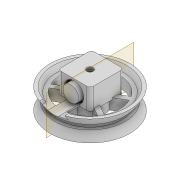
# Autodesk Inventor part: Primary_hinge
Saved by Autodesk Inventor 2022 (Build 260153000, 153)
## iProperties
Created: 2022-07-14
Part Number: Primary_hinge
Material: Generic
Document SubType Name: Modeling
Designer: dell
Density: 1 g/cm^3
Appearance: Default
Mass: 11.9893 g
Surface Area: 101.14 cm^2
Volume: 11.9893 cm^3
Author: dell
Autodesk Inventor part; units mm, degrees
ref_plane "XZ Plane" through (0, 0, 0) normal (0, 1, 0) x (-1, 0, 0)
ref_plane "XY Plane" through (0, 0, 0) normal (0, 0, 1) x (1, 0, 0)
sketch "Sketch1" plane through (0, 0, 0) normal (0, 0, 1) x (1, 0, 0)
  circle A0 centre (0, 0) radius 4.9
  circle A1 centre (0, 0) radius 6.1
  line L0 (-10.1, -7.1) -> (10.1, -7.1)
  line L1 (10.1, -7.1) -> (10.1, 7.1)
  line L2 (10.1, 7.1) -> (-10.1, 7.1)
  line L3 (-10.1, 7.1) -> (-10.1, -7.1)
  line L4 (-10.1, -7.1) -> (10.1, 7.1) construction
  line L5 (10.1, -7.1) -> (-10.1, 7.1) construction
  dimension "d0" = 9.8
  dimension "d1" = 12.2
  dimension "d3" = 4
  dimension "d4" = 1
  constraints: 12 end point, 2 centre point, 2 coincident, 2 midpoint, 2 parallel, 1 horizontal, 1 perpendicular
  measures "d0" diameter of A0
  measures "d1" diameter of A1
  measures "d3" distance edge to line of A1 L1
  measures "d4" distance edge to line of A1 L2
extrude "Extrusion1" add sketch "Sketch1" along normal blind 18
sketch "Sketch2" plane through (0, 0, 18) normal (0, 0, 1) x (1, 0, 0)
  circle A0 centre (0, 0) radius 4.9 projected
extrude "Extrusion2" add sketch "Sketch2" along normal blind 2
sketch "Sketch3" plane through (0, 0, 0) normal (0, 0, -1) x (-1, 0, 0)
  line L0 (-10.1, -7.1) -> (-10.1, 7.1) projected
  line L1 (10.1, -7.1) -> (-10.1, -7.1) projected
  line L2 (10.1, 7.1) -> (10.1, -7.1) projected
  line L3 (-10.1, 7.1) -> (10.1, 7.1) projected
  circle A0 centre (0, 0) radius 6.1 projected
extrude "Extrusion3" add sketch "Sketch3" along normal blind 3 contours L0 L3 L2 L1 | A0
ref_plane "Work Plane1" through (0, -7.1, 18) normal (-1, 0, 0) x (0, 0, 1)
sketch "Sketch6" plane through (-10.1, 7.1, 18) normal (0, 1, 0) x (1, 0, 0)
  line L0 (5.2, 18) -> (15, 18) projected
  line L1 (16.2, 18) -> (4, 18) projected
  line L2 (20.2, 0) -> (0, 0) projected
  line L3 (0, 21) -> (20.2, 21) projected
  line L4 (16.2, 0) -> (16.2, 18) projected
  line L5 (4, 0) -> (4, 18) projected
  circle A0 centre (10.1, 10) radius 2.05
  line L6 (0, 21) -> (0, 0) projected
  line L7 (20.2, 21) -> (20.2, 0) projected
  point P0 (10.1, 18)
  point P1 (10.1, 18)
  dimension "d49" = 4.1
  dimension "d50" = 10
  constraints: 1 centre point, 1 coincident, 1 midpoint, 1 vertical alignment
  measures "d49" diameter of A0
  measures "d50" distance from line of L2 A0.centre
extrude "Extrusion12" cut sketch "Sketch6" against normal blind 100 contours A0
fillet "Fillet5" radius 2 4 edges at (10.1, 0, 18) (-10.1, 0, 18) (10.1, 0, -3) (-10.1, 0, -3)
sketch "Sketch14" plane through (-8.1, -7.1, -3) normal (0, -1, 0) x (1, 0, 0)
  circle A0 centre (8.1, 11) radius 2.05 projected
  line L0 (8.1, 15.0415) -> (11.6, 13.0207)
  line L1 (11.6, 13.0207) -> (11.6, 8.9793)
  line L2 (11.6, 8.9793) -> (8.1, 6.9585)
  line L3 (8.1, 6.9585) -> (4.6, 8.9793)
  line L4 (4.6, 8.9793) -> (4.6, 13.0207)
  line L5 (4.6, 13.0207) -> (8.1, 15.0415)
  circle A1 centre (8.1, 11) radius 8
  point P0 (8.1, 3)
  dimension "d69" = 7
  dimension "d73" = 16
  constraints: 12 end point, 2 coincident, 1 centre point, 13 other
  measures "d69" distance between parallel lines of L1 L4
  measures "d73" diameter of A1
extrude "Extrusion14" add sketch "Sketch14" along normal blind 5 contours A1
sketch "Sketch15" plane through (0, -12.1, 8) normal (0, -1, 0) x (1, 0, 0)
  line L0 (3.4, -1) -> (4.8, -1)
  line L1 (4.8, -1) -> (4.8, -7.2415)
  line L2 (4.8, -7.2415) -> (3.4, -7.2415)
  line L3 (3.4, -7.2415) -> (3.4, -1)
  line L4 (3.4, -1) -> (4.8, -7.2415) construction
  line L5 (4.8, -1) -> (3.4, -7.2415) construction
  line L6 (0, 16.6) -> (0, -15.6) projected
  circle A0 centre (0, 0) radius 2.05 projected
  circle A1 centre (0, 0) radius 4.5
  circle A2 centre (0, 0) radius 8 projected
  line L7 (0, 4.0415) -> (3.5, 2.0207) projected
  line L8 (3.5, 2.0207) -> (3.5, -2.0207) projected
  line L9 (3.5, -2.0207) -> (0, -4.0415) projected
  line L10 (0, -4.0415) -> (-3.5, -2.0207) projected
  line L11 (-3.5, -2.0207) -> (-3.5, 2.0207) projected
  line L12 (-3.5, 2.0207) -> (0, 4.0415) projected
  circle A3 centre (0, 0) radius 8 projected
  line L13 (1.4, -7.8765) -> (3.4, -7.8765)
  line L14 (3.4, -7.8765) -> (3.4, -4.8765)
  line L15 (3.4, -4.8765) -> (1.4, -4.8765)
  line L16 (1.4, -4.8765) -> (1.4, -7.8765)
  line L17 (4.8, -6.4) -> (6.8, -6.4)
  line L18 (6.8, -6.4) -> (6.8, -2.4)
  line L19 (6.8, -2.4) -> (4.8, -2.4)
  line L20 (4.8, -2.4) -> (4.8, -6.4)
  line L21 (4.8, 1) -> (3.4, 1)
  line L22 (3.4, 1) -> (3.4, 7.2415)
  line L23 (3.4, 7.2415) -> (4.8, 7.2415)
  line L24 (4.8, 7.2415) -> (4.8, 1)
  line L25 (4.8, 1) -> (3.4, 7.2415) construction
  line L26 (3.4, 1) -> (4.8, 7.2415) construction
  line L27 (4.8, 6.4) -> (6.8, 6.4)
  line L28 (6.8, 6.4) -> (6.8, 3.4)
  line L29 (6.8, 3.4) -> (4.8, 3.4)
  line L30 (4.8, 3.4) -> (4.8, 6.4)
  line L31 (1.4, 8.7415) -> (3.4, 8.7415)
  line L32 (3.4, 8.7415) -> (3.4, 5.7415)
  line L33 (3.4, 5.7415) -> (1.4, 5.7415)
  line L34 (1.4, 5.7415) -> (1.4, 8.7415)
  point P0 (0, -8)
  point P1 (4.1, -4.1208)
  point P2 (4.8, -6.4)
  point P3 (6.8, -4.2143)
  point P4 (4.1, 4.1208)
  point P5 (4.8, 3.4)
  point P6 (6.8, 4.2143)
  point P7 (4.8, 6.4)
  point P8 (1.4, 7.8765)
  point P9 (4.8, 6.4)
  dimension "d74" = 4.1
  dimension "d75" = 1.4
  dimension "d76" = 9
  dimension "d77" = 1
  dimension "d78" = 2
  dimension "d79" = 3
  dimension "d80" = 2
  dimension "d81" = 4
  dimension "d84" = 1.4
  dimension "d85" = 1
  dimension "d86" = 4.1
  dimension "d87" = 2
  dimension "d88" = 3
  dimension "d89" = 2
  dimension "d90" = 3
  dimension "d97" = 1.5
  constraints: 56 end point, 12 parallel, 6 horizontal, 6 perpendicular, 4 midpoint, 4 point on circle, 4 point on line, 1 centre point, 1 coincident, 3 other
  measures "d74" distance from line of L6 point (4.1, -4.121)
  measures "d75" distance between parallel lines of L1 L3
  measures "d76" diameter of A1
  measures "d77" distance from line of A0.centre L0
  measures "d78" distance between parallel lines of L14 L16
  measures "d79" distance between parallel lines of L13 L15
  measures "d80" distance between parallel lines of L1 L18
  measures "d81" distance between parallel lines of L17 L19
  measures "d84" distance between parallel lines of L22 L24
  measures "d85" distance from line of A0.centre L21
  measures "d86" horizontal distance of A0.centre point (4.1, 4.121)
  measures "d87" distance of L28.end L29.end
  measures "d88" distance of L27.end L28.end
  measures "d89" distance of L31.start L31.end
  measures "d90" distance of L33.end L31.start
  measures "d97" distance between parallel lines of L23 L31
extrude "Extrusion15" add sketch "Sketch15" along normal blind 3 contours L33 L34 A2 L22 | L24 A2 L28 L29 | A2 L34 L31 L32 | L27 L28 A2
sketch "Sketch16" plane through (-3.5, -7.1, 5.9793) normal (0, -1, 0) x (1, 0, 0)
  line L0 (3.5, 6.0622) -> (0, 4.0415) projected
  line L1 (0, 4.0415) -> (0, 0) projected
  line L2 (0, 0) -> (3.5, -2.0207) projected
  line L3 (3.5, -2.0207) -> (7, 0) projected
  line L4 (7, 0) -> (7, 4.0415) projected
  line L5 (7, 4.0415) -> (3.5, 6.0622) projected
  circle A0 centre (3.5, 2.0207) radius 2.05 projected
  point P0 (3.5, -5.9793)
extrude "Extrusion16" add sketch "Sketch16" along normal blind 2.4
sketch "Sketch17" plane through (-8.1, -12.1, -3) normal (0, -1, 0) x (1, 0, 0)
  arc A0 (12.9, 17.4) -> (11.5, 18.2415) centre (8.1, 11) ccw projected
  circle A1 centre (8.1, 11) radius 25
  circle A2 centre (8.1, 11) radius 8
  point P0 (8.1, 3)
  point P1 (9.5, 18.8765)
  point P2 (9.5, 18.8765)
  point P3 (14.9, 15.2143)
  dimension "d94" = 17
  constraints: 2 centre point, 2 coincident, 1 concentric
  measures "d94" radial gap between concentric circles of A0 A1
extrude "Extrusion17" add sketch "Sketch17" against normal blind 2
sketch "Sketch19" plane through (0, 0, 18) normal (0, 0, 1) x (1, 0, 0)
  circle A0 centre (0, 0) radius 4.9 projected
  circle A1 centre (0, 0) radius 6.1 projected
  circle A2 centre (0, 0) radius 4.9 projected
sketch "Sketch18" plane through (-8.1, -7.1, -3) normal (0, -1, 0) x (1, 0, 0)
  circle A0 centre (8.1, 11) radius 25 projected
  arc A1 (-2, 2) -> (0, 0) centre (0, 2) ccw projected
  line L0 (16.2, 0) -> (0, 0) projected
  arc A2 (16.2, 0) -> (18.2, 2) centre (16.2, 2) ccw projected
  line L1 (18.2, 19) -> (18.2, 2) projected
  arc A3 (18.2, 19) -> (16.2, 21) centre (16.2, 19) ccw projected
  line L2 (0, 21) -> (16.2, 21) projected
  arc A4 (0, 21) -> (-2, 19) centre (0, 19) ccw projected
  line L3 (-2, 2) -> (-2, 19) projected
  circle A5 centre (8.1, 11) radius 8 projected
  point P0 (8.1, 3)
extrude "Extrusion18" add sketch "Sketch18" against normal blind 2 contours A0
extrude "Extrusion19" cut sketch "Sketch19" along normal blind 100
thicken "Thicken1" operation add thickness 12 both sides no extend neighbours yes toward (0.9967573, 0, -0.0804666) faces at (7.9741, -8.1, 7.3563)
sketch "Sketch20" plane through (0, -12.1, 8) normal (0, -1, 0) x (1, 0, 0)
  circle A0 centre (0, 0) radius 25 projected
  circle A1 centre (0, 0) radius 21
  point P0 (0, -8)
  dimension "d104" = 4
  constraints: 1 centre point
  measures "d104" radial gap between concentric circles of A0 A1
extrude "Extrusion20" add sketch "Sketch20" along normal blind 3
sketch "Sketch21" plane through (-8.1, -5.1, -3) normal (0, 1, 0) x (1, 0, 0)
  arc A0 (11.4466, -35.775) -> (4.7534, -35.775) centre (8.1, -11) ccw projected
  arc A1 (11.1556, -31.7765) -> (5.0444, -31.7765) centre (8.1, -11) ccw
  circle A2 centre (8.1, -11) radius 2.05 projected
  circle A3 centre (8.1, -11) radius 21
  circle A4 centre (8.1, -11) radius 21 projected
  line L0 (0.1, -30.4165) -> (0.1, -34.6854)
  line L1 (16.1, -30.4165) -> (16.1, -34.6854)
  point P0 (8.1, -3)
  point P1 (11.4466, -33.7552)
  point P2 (4.7534, -33.7552)
  point P3 (16.1, -30.4165)
  point P4 (18.1, -31.7123)
  point P5 (-1.9, -31.7123)
  point P6 (0.1, -30.4165)
  dimension "d107" = 4
  dimension "d108" = 8
  dimension "d109" = 8
  constraints: 6 point on circle, 4 end point, 2 centre point, 1 coincident, 1 concentric, 1 parallel, 1 vertical
  measures "d107" radial gap between concentric circles of A0 A1
  measures "d108" distance from line of A0.centre L1
  measures "d109" distance from line of A0.centre L0
extrude "Extrusion21" add sketch "Sketch21" along normal blind 3 contours L1 A1 L0 A0
chamfer "Chamfer1" distance 3 distance2 5 1 edges at (-25, -7.1, 8) measured on face at (-24.5, -7.1, 8)
chamfer "Chamfer2" distance 3 distance2 5 1 edges at (-25, -10.1, 8) measured on face at (-24.5, -10.1, 8)
chamfer "Chamfer3" distance 2 distance2 3 1 edges at (0, -2.1, -13) measured on face at (0, -2.1, -13.5)
chamfer "Chamfer4" distance 2 distance2 3 1 edges at (-21, -15.1, 8) measured on face at (-21.5, -15.1, 8)
sketch "Sketch22" plane through (0, -12.1, 8) normal (0, -1, 0) x (1, 0, 0)
  circle A0 centre (0.0592, 0.0061) radius 18.5
  circle A1 centre (0.0592, 0.0061) radius 9.5
  line L0 (-1.5, 18.4403) -> (-1.5, -18.4281)
  line L1 (1.5, -18.4377) -> (1.5, 18.4499)
  line L2 (0, 35) -> (0, -35) projected
  line L3 (-15.1257, -10.5613) -> (16.8033, 7.8729)
  line L4 (15.3116, 10.4758) -> (-16.634, -7.9681)
  line L5 (16.8033, -7.8607) -> (-15.1257, 10.5735)
  line L6 (-16.634, 7.9802) -> (15.3116, -10.4636)
  arc A2 (8, 21.7771) -> (3.3466, 22.9574) centre (0, 0) ccw projected
  line L7 (8, 21.7771) -> (8, 19.4165) projected
  arc A3 (-8, 19.4165) -> (8, 19.4165) centre (0, 0) ccw projected
  line L8 (-8, 19.4165) -> (-8, 21.7771) projected
  arc A4 (-3.3466, 22.9574) -> (-8, 21.7771) centre (0, 0) ccw projected
  line L9 (-3.3466, 22.9574) -> (-3.3466, 10) projected
  line L10 (-8.1, 10) -> (-3.3466, 10) projected
  arc A5 (-8.1, 10) -> (-10.1, 8) centre (-8.1, 8) ccw projected
  line L11 (-10.1, -9) -> (-10.1, 8) projected
  arc A6 (-10.1, -9) -> (-8.1, -11) centre (-8.1, -9) ccw projected
  line L12 (8.1, -11) -> (-8.1, -11) projected
  arc A7 (8.1, -11) -> (10.1, -9) centre (8.1, -9) ccw projected
  line L13 (10.1, 8) -> (10.1, -9) projected
  arc A8 (10.1, 8) -> (8.1, 10) centre (8.1, 8) ccw projected
  line L14 (3.3466, 10) -> (8.1, 10) projected
  line L15 (3.3466, 10) -> (3.3466, 22.9574) projected
  point P0 (0, -8)
  point P1 (16.8033, -7.8607)
  point P2 (-1.5, -9.3651)
  point P3 (8.9545, -3.3292)
  point P4 (15.3116, -10.4636)
  point P5 (7.4709, -5.9367)
  point P6 (-7.2769, -6.0298)
  point P7 (-16.634, -7.9681)
  point P8 (-8.7933, -3.4412)
  point P9 (-1.5, 9.3773)
  point P10 (-16.634, 7.9802)
  point P11 (1.5, 9.3962)
  point P12 (-8.7933, 3.4534)
  point P13 (10.1, -3.9906)
  point P14 (10.1, 7.4668)
  point P15 (-15.1257, 10.5735)
  point P16 (16.8033, 7.8729)
  point P17 (8.9545, 3.3414)
  point P18 (1.5, -9.384)
  point P19 (-10.1, 7.6719)
  point P20 (-1.5, -11)
  point P21 (-10.1, 4.2078)
  point P22 (-10.1, -7.6597)
  point P23 (-3.3466, 18.1899)
  point P24 (-10.0883, 8.2156)
  point P25 (10.0642, 8.3769)
  point P26 (3.3466, 18.2117)
  point P27 (1.5, -11)
  point P28 (10.1, 4.0027)
  point P29 (10.1, -7.4547)
  point P30 (-10.1, -4.1956)
  point P31 (0.1776, 1.7381)
  point P32 (0, 1.8407)
  point P33 (0, 1.6356)
  point P34 (0.1776, -1.726)
  point P35 (0, -1.6234)
  point P36 (0, -1.8285)
  point P37 (7.4709, 5.9489)
  point P38 (-7.2769, 6.042)
  dimension "d124" = 37
  dimension "d125" = 19
  dimension "d126" = 1.5
  dimension "d127" = 1.5
  dimension "d130" = 360
  constraints: 12 end point, 4 point on circle, 2 centre point, 1 coincident, 1 vertical, 19 other
  measures "d124" diameter of A0
  measures "d125" diameter of A1
  measures "d126" distance between parallel lines of L2 L1
  measures "d127" distance between parallel lines of L2 L0
extrude "Extrusion22" cut sketch "Sketch22" against normal blind 6 contours A0 L5 L13 L3 | L4 L13 A8 L14 L15 A0 | L13 L5 A1 L3 | A0 L1 L12 A7 L13 L6 | L15 L14 A8 L13 L4 A1 L1 A0 | L13 A7 L12 L1 A1 L6 | A0 L3 L11 A6 L12 L0 | L0 A1 L5 L11 A5 L10 L9 A0 | L4 L2 L5 | L3 L2 L6 | L12 A6 L11 L3 A1 L0 | L9 L10 A5 L11 L5 A0 | A0 L6 L11 L4 | L11 L6 A1 L4
extrude "Extrusion23" cut sketch "Sketch22" against normal blind 8 contours A0 L5 L13 L3 | L4 L13 A8 L14 L15 A0 | A0 L1 L12 A7 L13 L6 | A0 L3 L11 A6 L12 L0 | L3 L2 L6 | L9 L10 A5 L11 L5 A0 | A0 L6 L11 L4
body "Solid1"
